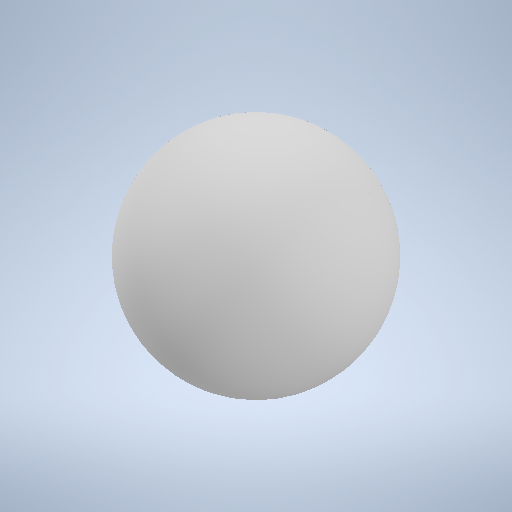
# Autodesk Inventor part: peca_007_001
Saved by Autodesk Inventor 2026 (Build 300175000, 175)
## iProperties
Created: 2025-03-26
Part Number: peca_007_001
Material: Generic
Document SubType Name: Modeling
Designer: Carlos Dias
Density: 1 g/cm^3
Appearance: Default
Author: Carlos Dias
Autodesk Inventor part; units mm, degrees
ref_plane "YZ Plane" through (0, 0, 0) normal (1, 0, 0) x (0, 1, 0)
ref_plane "XZ Plane" through (0, 0, 0) normal (0, 1, 0) x (-1, 0, 0)
ref_plane "XY Plane" through (0, 0, 0) normal (0, 0, 1) x (1, 0, 0)
sketch "Sketch2" plane through (0, 0, 0) normal (1, 0, 0) x (0, 1, 0)
  arc A0 (2, 0) -> (-2, 0) centre (0, 0) ccw
  line L0 (-2, 0) -> (2, 0)
  dimension "d1" = 2
  constraints: 2 end point, 2 horizontal alignment, 2 point on circle, 1 centre point, 1 coincident, 1 horizontal
  measures "d1" radius of A0
revolve "Revolution1" add sketch "Sketch2" angle 360 about axis through (0, -2, 0) along (0, 1, 0)
body "Solid1"
